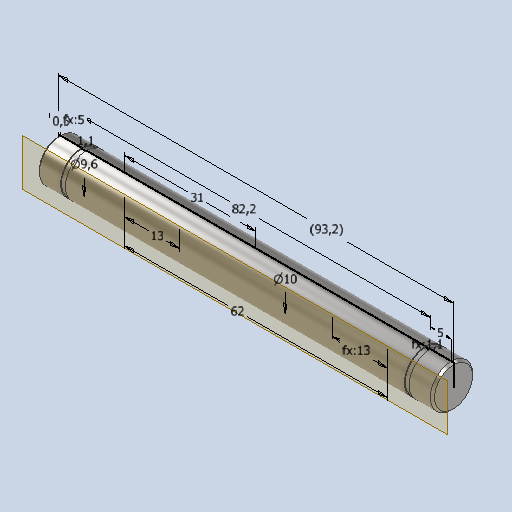
# Autodesk Inventor part: ParallelMecha_DrivenShaft
Saved by Autodesk Inventor 2024 (Build 280153000, 153)
## iProperties
Created: 2022-08-03
Part Number: ParallelMecha_DrivenShaft
Material: Edelstahl
Document SubType Name: Modeling
Designer: alexw
Density: 8 g/cm^3
Appearance: Halbpoliert
Mass: 56.0642 g
Surface Area: 30.9949 cm^2
Volume: 7.00803 cm^3
Author: alexw
Autodesk Inventor part; units mm, degrees
ref_plane "YZ Plane" through (0, 0, 0) normal (1, 0, 0) x (0, 1, 0)
ref_plane "XZ Plane" through (0, 0, 0) normal (0, 1, 0) x (-1, 0, 0)
sketch "Skizze1" plane through (0, 0, 0) normal (0, 0, 1) x (1, 0, 0)
  line L0 (0, 0) -> (0, 5)
  line L1 (93.2, 5) -> (93.2, 0)
  line L2 (93.2, 0) -> (0, 0)
  line L3 (5.5, 5) -> (5.5, 4.8)
  line L4 (5.5, 4.8) -> (6.6, 4.8)
  line L5 (6.6, 4.8) -> (6.6, 5)
  line L6 (0, 5) -> (5.5, 5)
  line L7 (86.6, 5) -> (86.6, 4.8)
  line L8 (86.6, 4.8) -> (87.7, 4.8)
  line L9 (87.7, 4.8) -> (87.7, 5)
  line L10 (6.6, 5) -> (86.6, 5)
  line L11 (87.7, 5) -> (93.2, 5)
  line L12 (46.6, 0) -> (46.6, 5) construction
  line L13 (0.5, 5) -> (0.5, 0) construction
  line L14 (92.7, 5) -> (92.7, 0) construction
  line L15 (15.6, 0) -> (15.6, 5) construction
  line L16 (77.6, 0) -> (77.6, 5) construction
  line L17 (28.6, 5) -> (28.6, 0) construction
  line L18 (64.6, 5) -> (64.6, 0) construction
  dimension "d2" = 10
  dimension "d3" = 9.6
  dimension "d4" = 1.1
  dimension "d6" = 1.1
  dimension "d8" = 82.2
  dimension "d9" = 5
  dimension "d10" = 5
  dimension "d11" = 0.5
  dimension "d12" = 93.2
  dimension "d16" = 31
  dimension "d17" = 62
  dimension "d18" = 13
  dimension "d19" = 13
  constraints: 36 end point, 13 perpendicular, 8 vertical, 6 point on line, 3 collinear, 1 midpoint, 10 other
  measures "d4" distance between parallel lines of L5 L3
  measures "d6" distance between parallel lines of L7 L9
  measures "d8" distance between parallel lines of L9 L3
  measures "d9" distance between parallel lines of L14 L9
  measures "d10" distance between parallel lines of L3 L13
  measures "d11" distance between parallel lines of L0 L13
  measures "d12" distance between parallel lines of L1 L0
  measures "d16" distance between parallel lines of L15 L12
  measures "d17" distance between parallel lines of L16 L15
  measures "d18" distance between parallel lines of L17 L15
  measures "d19" distance between parallel lines of L16 L18
revolve "Umdrehung1" add sketch "Skizze1" angle 360 about axis through (93.2, 0, 0) along (-1, 0, 0)
sketch "Skizze2" plane through (46.6, 0, 5) normal (0, 0, 1) x (1, 0, 0)
  line L0 (-31, 0) -> (-31, 5) construction
  line L1 (-18, 5) -> (-18, 0) construction
  line L2 (18, 5) -> (18, 0) construction
  line L3 (31, 0) -> (31, 5) construction
  line L4 (-31, 5) -> (-18, 5)
  line L5 (-18, 5) -> (-18, -5)
  line L6 (-18, -5) -> (-31, -5)
  line L7 (-31, -5) -> (-31, 5)
  line L8 (18, 5) -> (31, 5)
  line L9 (31, 5) -> (31, -5)
  line L10 (31, -5) -> (18, -5)
  line L11 (18, -5) -> (18, 5)
  point P0 (-46.6, 0)
  dimension "d20" = 10
  dimension "d21" = 10
  constraints: 16 end point, 4 parallel, 2 collinear, 2 horizontal, 2 perpendicular
  measures "d20" distance between parallel lines of L4 L6
  measures "d21" distance between parallel lines of L8 L10
chamfer "Fase1" distance 0.5 angle 45 2 edges at (0, -5, 0) (93.2, -5, 0)
ref_plane "Arbeitsebene1" through (46.6, 0, 5) normal (0, 0, 1) x (1, 0, 0)
equation "\"d20\" = d2"
equation "\"d21\" = d20"
equation "\"d6\" = d4"
equation "\"d10\" = d9"
equation "\"d19\" = d18"
